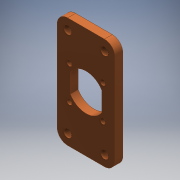
# Autodesk Inventor part: motor_plate
Saved by Autodesk Inventor 2016 (Build 200138000, 138)
## iProperties
Created: 2015-12-08
Part Number: motor_plate
Material: Generic
Document SubType Name: Modeling
Designer: lk8187
Density: 1 g/cm^3
Appearance: Smooth - Dark Brown
Author: lk8187
Autodesk Inventor part; units mm, degrees
ref_plane "YZ Plane" through (0, 0, 0) normal (1, 0, 0) x (0, 1, 0)
ref_plane "XZ Plane" through (0, 0, 0) normal (0, 1, 0) x (-1, 0, 0)
ref_plane "XY Plane" through (0, 0, 0) normal (0, 0, 1) x (1, 0, 0)
sketch "Sketch1" plane through (0, 0, 0) normal (0, 1, 0) x (-1, 0, 0)
  line L0 (7, 21) -> (-7, 21)
  line L1 (-11, 17) -> (-11, -17)
  line L2 (-7, -21) -> (7, -21)
  line L3 (11, -17) -> (11, 17)
  line L4 (6, 3.6056) -> (6, -3.6056)
  line L5 (-6, -3.6056) -> (-6, 3.6056)
  line L6 (6.364, 6.364) -> (-6.364, 6.364) construction
  line L7 (-6.364, 6.364) -> (-6.364, -6.364) construction
  line L8 (-6.364, -6.364) -> (6.364, -6.364) construction
  line L9 (6.364, -6.364) -> (6.364, 6.364) construction
  arc A0 (-6, -3.6056) -> (6, -3.6056) centre (0, 0) ccw
  arc A1 (6, 3.6056) -> (-6, 3.6056) centre (0, 0) ccw
  arc A2 (-11, -17) -> (-7, -21) centre (-7, -17) ccw
  arc A3 (-7, 21) -> (-11, 17) centre (-7, 17) ccw
  arc A4 (11, 17) -> (7, 21) centre (7, 17) ccw
  arc A5 (7, -21) -> (11, -17) centre (7, -17) ccw
  point P0 (0, -21)
  point P1 (0, -7)
  point P2 (6.364, 0)
  point P3 (11, 0)
  point P4 (6, 0)
  point P5 (0, -6.364)
  dimension "d0" = 7
  dimension "d1" = 12
  dimension "d2" = 18
  dimension "d3" = 22
  dimension "d4" = 42
  dimension "d5" = 4
  constraints: 20 end point, 13 point on circle, 9 coincident, 8 tangent, 6 centre point, 5 midpoint, 5 parallel, 3 equal radius, 3 horizontal alignment, 3 perpendicular, 3 vertical alignment, 2 horizontal, 1 vertical
  measures "d0" radius of A0
  measures "d1" distance between parallel lines of L4 L5
  measures "d2" distance of L6.start L7.end
  measures "d3" distance between parallel lines of L3 L1
  measures "d4" distance between parallel lines of L0 L2
  measures "d5" radius of A2
extrude "Extrusion1" add sketch "Sketch1" against normal blind 3
hole "Hole1" at (-7, 0, 17) at (7, 0, 17) at (7, 0, -17) at (-7, 0, -17) direction (0, -1, 0) diameter 3 end through all
hole "Hole2" at (-6.364, 0, -6.364) at (6.364, 0, -6.364) at (6.364, 0, 6.364) at (-6.364, 0, 6.364) direction (0, -1, 0) diameter 2 end through all
body "Solid1"
